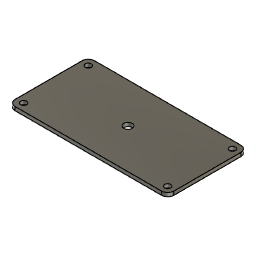
Platform_ middle (Autodesk Fusion 360 design; units mm, degrees)
Autodesk Fusion 360 part; units mm, degrees
sketch "Sketch1" plane through (0, 0, 0) normal (0, 0, 1) x (1, 0, 0)
  line L0 (-60, 32.5) -> (60, 32.5)
  line L1 (65, 27.5) -> (65, -27.5)
  line L2 (60, -32.5) -> (-60, -32.5)
  line L3 (-65, -27.5) -> (-65, 27.5)
  arc A0 (-60, 32.5) -> (-65, 27.5) centre (-60, 27.5) ccw
  arc A1 (-65, -27.5) -> (-60, -32.5) centre (-60, -27.5) ccw
  arc A2 (65, 27.5) -> (60, 32.5) centre (60, 27.5) ccw
  arc A3 (60, -32.5) -> (65, -27.5) centre (60, -27.5) ccw
  circle A4 centre (-59, 26.5) radius 2.5
  circle A5 centre (-59, -26.5) radius 2.5
  circle A6 centre (59, 26.5) radius 2.5
  circle A7 centre (59, -26.5) radius 2.5
  circle A8 centre (0, 0) radius 3.5
  dimension "d1" = 65
  dimension "d2" = 65
  dimension "d3" = 32.5
  dimension "d4" = 32.5
  dimension "d5" = 5
  dimension "d6" = 5
  dimension "d7" = 5
  dimension "d8" = 5
  dimension "d9" = 5
  dimension "d10" = 6
  dimension "d11" = 6
  dimension "d12" = 5
  dimension "d13" = 6
  dimension "d14" = 6
  dimension "d15" = 5
  dimension "d16" = 6
  dimension "d17" = 6
  dimension "d18" = 5
  dimension "d19" = 6
  dimension "d20" = 6
  dimension "d21" = 7
  constraint horizontal L0
  constraint vertical L1
  constraint horizontal L2
  constraint vertical L3
  constraint tangent L0 A0
  constraint tangent L3 A0
  constraint tangent L2 A1
  constraint tangent L3 A1
  constraint tangent L0 A2
  constraint tangent L1 A2
  constraint tangent L1 A3
  constraint tangent L2 A3
  constraint coincident A8.centre origin
  measures "d1" distance of A8.centre L3
  measures "d2" distance of A8.centre L1
  measures "d3" distance of A8.centre L0
  measures "d4" distance of A8.centre L2
  measures "d5" radius of A0
  measures "d6" radius of A1
  measures "d7" radius of A2
  measures "d8" radius of A3
  measures "d9" diameter of A4
  measures "d10" distance of L0 A4.centre
  measures "d11" distance of L3 A4.centre
  measures "d12" diameter of A5
  measures "d13" distance of L2 A5.centre
  measures "d14" distance of L3 A5.centre
  measures "d15" diameter of A6
  measures "d16" distance of L0 A6.centre
  measures "d17" distance of L1 A6.centre
  measures "d18" diameter of A7
  measures "d19" distance of L1 A7.centre
  measures "d20" distance of L2 A7.centre
  measures "d21" diameter of A8
extrude "Extrude1" add sketch "Sketch1" along normal blind 3
equation "d2 = d1"
equation "d3 = ( 65 / 2 ) * 1 mm"
equation "d4 = d3"
equation "d6 = d5"
equation "d7 = d5"
equation "d8 = d5"
equation "d11 = d10"
equation "d12 = d9"
equation "d13 = d10"
equation "d14 = d10"
equation "d15 = d9"
equation "d16 = d10"
equation "d17 = d10"
equation "d18 = d9"
equation "d19 = d10"
equation "d20 = d10"
